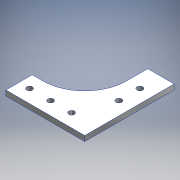
# Autodesk Inventor part: Brace
Saved by Autodesk Inventor 2019.4 (Build 234330000, 330)
## iProperties
Created: 2019-12-11
Part Number: Brace
Material: Aluminum 6061
Document SubType Name: Modeling
Designer: Mark
Density: 2.7 g/cm^3
Appearance: Aluminum - Flat
Mass: 74.3871 g
Surface Area: 139.413 cm^2
Volume: 27.5508 cm^3
Author: Mark
Autodesk Inventor part; units mm, degrees
ref_plane "YZ Plane" through (0, 0, 0) normal (1, 0, 0) x (0, 1, 0)
ref_plane "XZ Plane" through (0, 0, 0) normal (0, 1, 0) x (-1, 0, 0)
ref_plane "XY Plane" through (0, 0, 0) normal (0, 0, 1) x (1, 0, 0)
sketch "Sketch1" plane through (0, 0, 0) normal (0, 1, 0) x (-1, 0, 0)
  line L0 (0, 0) -> (15, 0)
  line L1 (15, 0) -> (15, -60)
  line L2 (15, -60) -> (0, -60)
  line L3 (0, -60) -> (0, 0)
  circle A0 centre (7.5, -40) radius 2.75
  line L4 (0, 0) -> (-105, 0)
  line L5 (-105, 0) -> (-105, -25)
  line L6 (-105, -25) -> (0, -25)
  line L7 (0, -25) -> (0, 0)
  line L8 (-105, -25) -> (-80, -25)
  line L9 (-80, -25) -> (-80, -85)
  line L10 (-80, -85) -> (-105, -85)
  line L11 (-105, -85) -> (-105, -25)
  circle A1 centre (7.5, -20) radius 2.75
  circle A2 centre (-20, -12.5) radius 2.75
  circle A3 centre (-40, -12.5) radius 2.75
  circle A4 centre (-60, -12.5) radius 2.75
  circle A5 centre (-80, -12.5) radius 2.75
  circle A6 centre (-92.5, -45) radius 2.75
  circle A7 centre (-92.5, -65) radius 2.75
  line L12 (-30, -25) -> (-30, 0)
  dimension "d0" = 15
  dimension "d1" = 60
  dimension "d2" = 5.5
  dimension "d3" = 40
  dimension "d4" = 7.5
  dimension "d5" = 105
  dimension "d6" = 25
  dimension "d7" = 60
  dimension "d8" = 25
  dimension "d9" = 5.5
  dimension "d10" = 7.5
  dimension "d11" = 20
  dimension "d12" = 5.5
  dimension "d13" = 12.5
  dimension "d14" = 20
  dimension "d17" = 20
  dimension "d22" = 5.5
  dimension "d23" = 5.5
  dimension "d24" = 12.5
  dimension "d25" = 12.5
  dimension "d26" = 20
  dimension "d27" = 20
  dimension "d31" = 10
  constraints: 26 end point, 8 centre point, 6 parallel, 4 horizontal, 4 perpendicular, 2 point on line, 6 other
  measures "d0" distance of L1.end L2.end
  measures "d1" distance of L0.end L1.end
  measures "d2" diameter of A0
  measures "d3" distance from line of L0 A0.centre
  measures "d4" distance from line of L3 A0.centre
  measures "d5" distance of L6.end L5.end
  measures "d6" distance of L5.end L4.end
  measures "d7" distance of L8.end L9.end
  measures "d8" distance of L9.end L10.end
  measures "d9" diameter of A1
  measures "d10" distance from line of L7 A1.centre
  measures "d11" distance from line of L0 A1.centre
  measures "d12" diameter of A2
  measures "d13" distance from line of L4 A2.centre
  measures "d14" distance from line of L3 A2.centre
  measures "d17" distance of A2.centre A3.centre
  measures "d22" diameter of A6
  measures "d23" diameter of A7
  measures "d24" distance from line of L11 A6.centre
  measures "d25" distance from line of L11 A7.centre
  measures "d26" distance from line of L10 A7.centre
  measures "d27" distance from line of L8 A6.centre
  measures "d31" distance from line of A3.centre L12
extrude "Extrusion1" add sketch "Sketch1" along normal blind 5 contours L12 L6 L5 L4 | L9 L10 L11 L6
fillet "Fillet1" radius 40 1 edges at (80, 2.5, -25)
body "Solid1"
